Autodesk Inventor part; units mm, degrees
(part 2 of 2)
sketch "Sketch8" plane through (0, 0, 0) normal (0, 0, -1) x (-1, 0, 0)
  circle A0 centre (-9.222618, -23.066498) radius 1.25
  arc A1 (-6.852288, -24.648912) -> (-5.454999, -24.922583) centre (-5.454876, -21.21803) ccw
  arc A2 (-7.079113, -24.944764) -> (-6.852288, -24.648912) centre (-9.222618, -23.066498) ccw
  arc A3 (-6.452085, -26.223102) -> (-7.079113, -24.944764) centre (-10.029598, -27.184931) ccw
  arc A4 (-6.887807, -26.557724) -> (-6.452085, -26.223102) centre (-9.222618, -23.066498) ccw
  arc A5 (-7.961059, -25.622074) -> (-6.887807, -26.557724) centre (-5.035423, -23.349549) ccw
  arc A6 (-8.305421, -25.764877) -> (-7.961059, -25.622074) centre (-9.222618, -23.066498) ccw
  arc A7 (-8.401568, -27.185463) -> (-8.305421, -25.764877) centre (-11.9807, -26.229676) ccw
  arc A8 (-8.946225, -27.257393) -> (-8.401568, -27.185463) centre (-9.222618, -23.066498) ccw
  arc A9 (-9.407864, -25.910471) -> (-8.946225, -27.257393) centre (-5.737927, -25.405224) ccw
  arc A10 (-9.777492, -25.861961) -> (-9.407864, -25.910471) centre (-9.222618, -23.066498) ccw
  arc A11 (-10.571051, -27.044151) -> (-9.777492, -25.861961) centre (-13.192776, -24.42685) ccw
  arc A12 (-11.078703, -26.834116) -> (-10.571051, -27.044151) centre (-9.222618, -23.066498) ccw
  arc A13 (-10.805032, -25.436828) -> (-11.078703, -26.834116) centre (-7.37415, -26.83424) ccw
  arc A14 (-11.100884, -25.210003) -> (-10.805032, -25.436828) centre (-9.222618, -23.066498) ccw
  arc A15 (-12.379222, -25.83703) -> (-11.100884, -25.210003) centre (-13.341052, -22.259518) ccw
  arc A16 (-12.713844, -25.401308) -> (-12.379222, -25.83703) centre (-9.222618, -23.066498) ccw
  arc A17 (-11.778194, -24.328057) -> (-12.713844, -25.401308) centre (-9.505669, -27.253692) ccw
  arc A18 (-11.920997, -23.983694) -> (-11.778194, -24.328057) centre (-9.222618, -23.066498) ccw
  arc A19 (-13.341583, -23.887547) -> (-11.920997, -23.983694) centre (-12.385796, -20.308416) ccw
  arc A20 (-13.413513, -23.34289) -> (-13.341583, -23.887547) centre (-9.222618, -23.066498) ccw
  arc A21 (-12.066591, -22.881252) -> (-13.413513, -23.34289) centre (-11.561344, -26.551189) ccw
  arc A22 (-12.018081, -22.511624) -> (-12.066591, -22.881252) centre (-9.222618, -23.066498) ccw
  arc A23 (-13.200271, -21.718065) -> (-12.018081, -22.511624) centre (-10.58297, -19.096339) ccw
  arc A24 (-12.990236, -21.210413) -> (-13.200271, -21.718065) centre (-9.222618, -23.066498) ccw
  arc A25 (-11.592948, -21.484083) -> (-12.990236, -21.210413) centre (-12.99036, -24.914965) ccw
  arc A26 (-11.366123, -21.188231) -> (-11.592948, -21.484083) centre (-9.222618, -23.066498) ccw
  arc A27 (-11.99315, -19.909894) -> (-11.366123, -21.188231) centre (-8.415638, -18.948064) ccw
  arc A28 (-11.557428, -19.575272) -> (-11.99315, -19.909894) centre (-9.222618, -23.066498) ccw
  arc A29 (-10.484177, -20.510922) -> (-11.557428, -19.575272) centre (-13.409812, -22.783446) ccw
  arc A30 (-10.139814, -20.368118) -> (-10.484177, -20.510922) centre (-9.222618, -23.066498) ccw
  arc A31 (-10.043667, -18.947532) -> (-10.139814, -20.368118) centre (-6.464536, -19.903319) ccw
  arc A32 (-9.49901, -18.875602) -> (-10.043667, -18.947532) centre (-9.222618, -23.066498) ccw
  arc A33 (-9.037372, -20.222524) -> (-9.49901, -18.875602) centre (-12.707309, -20.727771) ccw
  arc A34 (-8.667744, -20.271034) -> (-9.037372, -20.222524) centre (-9.222618, -23.066498) ccw
  arc A35 (-7.874185, -19.088844) -> (-8.667744, -20.271034) centre (-5.252459, -21.706146) ccw
  arc A36 (-7.366533, -19.298879) -> (-7.874185, -19.088844) centre (-9.222618, -23.066498) ccw
  arc A37 (-7.640203, -20.696167) -> (-7.366533, -19.298879) centre (-11.071085, -19.298755) ccw
  arc A38 (-7.344351, -20.922993) -> (-7.640203, -20.696167) centre (-9.222618, -23.066498) ccw
  arc A39 (-6.066014, -20.295965) -> (-7.344351, -20.922993) centre (-5.104184, -23.873478) ccw
  arc A40 (-5.731392, -20.731687) -> (-6.066014, -20.295965) centre (-9.222618, -23.066498) ccw
  arc A41 (-6.667042, -21.804939) -> (-5.731392, -20.731687) centre (-8.939567, -18.879303) ccw
  arc A42 (-6.524238, -22.149301) -> (-6.667042, -21.804939) centre (-9.222618, -23.066498) ccw
  arc A43 (-5.103652, -22.245448) -> (-6.524238, -22.149301) centre (-6.059439, -25.82458) ccw
  arc A44 (-5.031722, -22.790105) -> (-5.103652, -22.245448) centre (-9.222618, -23.066498) ccw
  arc A45 (-6.378644, -23.251744) -> (-5.031722, -22.790105) centre (-6.883891, -19.581807) ccw
  arc A46 (-6.427154, -23.621372) -> (-6.378644, -23.251744) centre (-9.222618, -23.066498) ccw
  arc A47 (-5.244964, -24.414931) -> (-6.427154, -23.621372) centre (-7.862266, -27.036656) ccw
  arc A48 (-5.454999, -24.922583) -> (-5.244964, -24.414931) centre (-9.222618, -23.066498) ccw
  circle A49 centre (-9.222618, -23.066498) radius 4.2
  circle A50 centre (-9.222618, -23.066498) radius 4.6
  point P0 (0, 0)
  dimension "d138" = 0.4
  constraints: 1 centre point, 1 coincident, 3 other
extrude "Extrusion10" add sketch "Sketch8" against normal blind 1.6 contours A2 A3 A4 A5 A6 A7 A8 A9 A10 A11 A12 A13 A14 A15 A16 A17 A18 A19 A20 A21 A22 A23 A24 A25 A26 A27 A28 A29 A30 A31 A32 A33 A34 A35 A36 A37 A38 A39 A40 A41 A42 A43 A44 A45 A46 A47 A48 A1 | A1 A49 A3 A2 | A47 A46 A45 A49 | A49 A7 A6 A5 | A43 A42 A41 A49 | A49 A11 A10 A9 | A39 A38 A37 A49 | A49 A15 A14 A13 | A35 A34 A33 A49 | A49 A19 A18 A17 | A31 A30 A29 A49 | A49 A23 A22 A21 | A27 A26 A25 A49 | A50
fillet "Fillet1" radius 1 5 edges at (1.9609, -60.1053, 2) (5.9625, -57.7949, 2) (8.4625, -62.125, 2) (4.4609, -64.4354, 2) (20.9375, -49.1491, 2)
sketch "Sketch10" plane through (0, 0, 9.3) normal (0, 0, 1) x (1, 0, 0)
  arc A0 (2, -23.367949) -> (-1, -25.1) centre (1, -25.1) ccw
  line L0 (-1, -33.180447) -> (-1, -25.1)
  spline S0 degree 2 poles (-1, -33.180447) (0.437273, -35.168536) (-1, -37.156626) knots 0 0 0 1 1 1 weights 1 1.44736842 1 construction
  line L1 (-1, -45.237072) -> (-1, -37.156626)
  line L2 (23.1, -65.837072) -> (0, -65.837072)
  line L3 (23.1, -6.5) -> (23.1, -65.837072)
  line L4 (27.4, -6.5) -> (23.1, -6.5)
  line L5 (27.4, 0) -> (27.4, -6.5)
  line L6 (0, 0) -> (27.4, 0)
  line L7 (0, -1) -> (0, 0)
  line L8 (2.5, -1) -> (0, -1)
  line L9 (2.5, -17.5) -> (2.5, -1)
  line L10 (0, -17.5) -> (2.5, -17.5)
  line L11 (0, -65.837072) -> (0, -17.5)
  arc A1 (4.054242, -29.688272) -> (16.938443, -26.387046) centre (12.35, -35.272213) ccw
  arc A2 (9.70004, -14.680076) -> (4.054242, -29.688272) centre (9.222618, -23.066498) ccw
  arc A3 (16.718073, -19.274645) -> (9.70004, -14.680076) centre (14.7, -14.7) ccw
  arc A4 (16.938443, -26.387046) -> (16.718073, -19.274645) centre (9.222618, -23.066498) ccw
  circle A5 centre (1.4, -30.091255) radius 0.6
  circle A6 centre (1.4, -41.171175) radius 0.6
  circle A7 centre (1.4, -30.091255) radius 2.113828
  circle A8 centre (1.4, -41.171175) radius 2.437856
  circle A9 centre (4, -46.509539) radius 3.5
  arc A10 (4.054242, -29.688272) -> (16.938443, -26.387046) centre (12.35, -35.272213) ccw
  arc A11 (9.70004, -14.680076) -> (4.054242, -29.688272) centre (9.222618, -23.066498) ccw
  circle A12 centre (9.043146, -9.043146) radius 2.25
  circle A13 centre (20.356854, -20.356854) radius 2.25
  arc A14 (-1, -45.237072) -> (2, -46.969123) centre (1, -45.237072) ccw
  spline S1 degree 3 poles (3, -25.1) (3, -24.918932) (2.974149, -24.721818) (2.859633, -24.337077) (2.770851, -24.149343) (2.583999, -23.871436) (2.486925, -23.753405) (2.26049, -23.539413) (2.130887, -23.443517) (2, -23.367949) knots 0 0 0 0 0.29735014 0.29735014 0.59470027 0.59470027 0.79735014 0.79735014 1 1 1 1
  spline S2 degree 3 poles (2, -46.969123) (2.144805, -46.88552) (2.285887, -46.778364) (2.528279, -46.538397) (2.629848, -46.405654) (2.897307, -45.967482) (3, -45.573174) (3, -45.237072) knots 0 0 0 0 0.2241219 0.2241219 0.4482438 0.4482438 1 1 1 1
  line L12 (3, -25.1) -> (3, -45.237072)
  circle A15 centre (4, -46.509539) radius 1.2295
  point P0 (0, 0)
  point P1 (19.495918, -28.276795)
  dimension "d145" = 1.2
  dimension "d146" = 1.2
  dimension "d147" = 4.22766
  dimension "d148" = 4.87571
  dimension "d149" = 7
  dimension "d226" = 0.8
  dimension "d227" = 1
  dimension "d228" = 0.8
  dimension "d229" = 1
  constraints: 5 centre point, 4 tangent, 3 coincident, 2 end point, 1 vertical
  measures "d145" diameter of A5
  measures "d146" diameter of A6
  measures "d147" diameter of A7
  measures "d148" diameter of A8
  measures "d149" diameter of A9
  measures "d226" distance edge to line of A5 L11
  measures "d227" distance edge to line of A5 L12
  measures "d228" distance edge to line of A6 L11
  measures "d229" distance edge to line of A6 L12
hole "Hole7" at (1.4, -30.091255, 9.3) at (1.4, -41.171175, 9.3) direction (0, 0, -1) diameter 1.4 end through all
sketch "Sketch11" plane through (2.5, -17.5, 0) normal (-1, 0, 0) x (0, 0, 1)
  circle A0 centre (6, 7) radius 1.25 projected
  point P0 (0, 17.5)
hole "Hole8" at (2.5, -10.5, 6) direction (1, 0, 0) diameter 2.013 depth 8 thread size "M2.5x0.45" class "6H" standard "ISO Metric profile"
sketch "Sketch13" plane through (0, 0, 3.1) normal (0, 0, 1) x (1, 0, 0)
  arc A0 (6.782075, -26.965696) -> (13.237489, -25.311672) centre (12.35, -35.272213) ccw
  arc A1 (6.782075, -26.965696) -> (13.237489, -25.311672) centre (9.222618, -23.066498) ccw
  circle A2 centre (12.35, -35.272213) radius 5
  circle A3 centre (14.7, -14.7) radius 14
  circle A4 centre (14.7, -55.637072) radius 14
  circle A5 centre (18.362153, -30.788463) radius 2.5
  circle A6 centre (18.490592, -39.578386) radius 2.5
  circle A7 centre (6.124853, -31.089206) radius 2.5
  circle A8 centre (7.351555, -40.863773) radius 2.5
  point P0 (0, 0)
  dimension "d174" = 5
  dimension "d175" = 5
  dimension "d176" = 5
  dimension "d177" = 5
  dimension "d178" = 1.5
  constraints: 7 tangent, 4 centre point
  measures "d174" diameter of A5
  measures "d175" diameter of A6
  measures "d176" diameter of A8
  measures "d177" diameter of A7
hole "Hole10" at (18.362153, -30.788463, 3.1) at (18.490592, -39.578386, 3.1) at (7.351555, -40.863773, 3.1) at (6.124853, -31.089206, 3.1) direction (0, 0, -1) diameter 2.9 end through all counterbore diameter 5 counterbore depth 1.1 clearance for "Countersunk Flat Head Screw ISO 2009/7046" size "M2.5" standard "ISO"
sketch "Sketch14" plane through (0, 0, 3.1) normal (0, 0, 1) x (1, 0, 0)
  arc A0 (8.199902, -32.483542) -> (4.049804, -29.694871) centre (6.124853, -31.089206) ccw
  arc A1 (16.358102, -32.283046) -> (8.199902, -32.483542) centre (12.35, -35.272213) ccw
  arc A2 (20.366204, -29.293879) -> (16.358102, -32.283046) centre (18.362153, -30.788463) ccw
  arc A3 (20.366204, -29.293879) -> (13.237489, -25.311672) centre (12.35, -35.272213) ccw
  arc A4 (6.782075, -26.965696) -> (13.237489, -25.311672) centre (9.222618, -23.066498) ccw
  arc A5 (6.782075, -26.965696) -> (4.049804, -29.694871) centre (12.35, -35.272213) ccw
  arc A6 (20.537456, -41.013777) -> (16.443728, -38.142995) centre (18.490592, -39.578386) ccw
  arc A7 (20.537456, -41.013777) -> (20.366204, -29.293879) centre (12.35, -35.272213) ccw
  arc A8 (16.358102, -32.283046) -> (20.366204, -29.293879) centre (18.362153, -30.788463) ccw
  arc A9 (16.443728, -38.142995) -> (16.358102, -32.283046) centre (12.35, -35.272213) ccw
  arc A10 (5.685407, -42.727627) -> (9.017703, -38.99992) centre (7.351555, -40.863773) ccw
  arc A11 (5.685407, -42.727627) -> (20.537456, -41.013777) centre (12.35, -35.272213) ccw
  arc A12 (16.443728, -38.142995) -> (20.537456, -41.013777) centre (18.490592, -39.578386) ccw
  arc A13 (9.017703, -38.99992) -> (16.443728, -38.142995) centre (12.35, -35.272213) ccw
  arc A14 (4.049804, -29.694871) -> (8.199902, -32.483542) centre (6.124853, -31.089206) ccw
  arc A15 (4.049804, -29.694871) -> (5.685407, -42.727627) centre (12.35, -35.272213) ccw
  arc A16 (9.017703, -38.99992) -> (5.685407, -42.727627) centre (7.351555, -40.863773) ccw
  arc A17 (8.199902, -32.483542) -> (9.017703, -38.99992) centre (12.35, -35.272213) ccw
  line L0 (16.28503, -29.39722) -> (15.132486, -31.117965)
  line L1 (19.103243, -33.176095) -> (17.125264, -33.790033)
  line L2 (15.252677, -39.343388) -> (16.455005, -41.029724)
  circle A18 centre (12.35, -35.272213) radius 5
  line L3 (10.45085, -39.897494) -> (9.664196, -41.813348)
  line L4 (7.965712, -37.675963) -> (6.14968, -38.671629)
  line L5 (9.366807, -31.259662) -> (8.131128, -29.59761)
  line L6 (5.501944, -33.51036) -> (7.507693, -34.026395)
  line L7 (17.166531, -36.614236) -> (19.161604, -37.17012)
  arc A19 (4.049804, -29.694871) -> (8.199902, -32.483542) centre (6.124853, -31.089206) ccw
  arc A20 (8.199902, -32.483542) -> (4.049804, -29.694871) centre (6.124853, -31.089206) ccw
  arc A21 (9.017703, -38.99992) -> (5.685407, -42.727627) centre (7.351555, -40.863773) ccw
  arc A22 (5.685407, -42.727627) -> (9.017703, -38.99992) centre (7.351555, -40.863773) ccw
  arc A23 (9.017703, -38.99992) -> (16.443728, -38.142995) centre (12.35, -35.272213) ccw
  arc A24 (16.443728, -38.142995) -> (20.537456, -41.013777) centre (18.490592, -39.578386) ccw
  arc A25 (16.358102, -32.283046) -> (20.366204, -29.293879) centre (18.362153, -30.788463) ccw
  arc A26 (16.358102, -32.283046) -> (8.199902, -32.483542) centre (12.35, -35.272213) ccw
  point P0 (0, 0)
  point P1 (16.358102, -32.283046)
  point P2 (16.358102, -32.283046)
  point P3 (16.358102, -32.283046)
  point P4 (16.358102, -32.283046)
  point P5 (16.443728, -38.142995)
  point P6 (16.443728, -38.142995)
  point P7 (16.443728, -38.142995)
  point P8 (16.443728, -38.142995)
  constraints: 18 point on circle, 16 end point, 8 tangent, 2 line through centre, 12 other
extrude "Extrusion12" cut sketch "Sketch14" against normal up to surface (1.1 mm away) contours A0 L5 A1 | A17 L6 A14 | L0 A2 A1 | A17 A16 L4 | A8 L1 A9 | A13 L3 A10 | A6 A9 L7 | L2 A13 A12
sketch "Sketch15" plane through (0, 0, 0) normal (0, 1, 0) x (1, 0, 0)
  line L0 (27.4, 0) -> (0, 0) projected
  line L1 (0, 0) -> (0, -9.3) projected
  line L2 (0, -9.3) -> (27.4, -9.3) projected
  line L3 (27.4, 0) -> (27.4, -9.3) projected
  line L4 (27.4, 0) -> (0, 0) projected
  line L5 (23.1, 0) -> (23.1, -9.3)
  line L6 (3, -9.3) -> (3, 0)
  line L7 (0, 0) -> (0, -9.3) projected
  circle A0 centre (18.075, -3.25) radius 3.25
  circle A1 centre (8.025, -3.25) radius 3.25
  line L8 (13.05, 0) -> (13.05, -9.3)
  dimension "d195" = 4.3
  dimension "d196" = 3
  dimension "d197" = 6.5
  dimension "d198" = 6.5
  dimension "d202" = 5.025
  dimension "d203" = 5.025
  dimension "d206" = 10.05
  dimension "d207" = 10.05
  dimension "d208" = 5.025
  dimension "d209" = 5.025
  constraints: 6 end point, 6 point on line, 2 centre point, 2 perpendicular, 2 tangent, 1 parallel
  measures "d195" distance between parallel lines of L3 L5
  measures "d196" distance between parallel lines of L1 L6
  measures "d197" diameter of A0
  measures "d198" diameter of A1
  measures "d202" distance from line of A0.centre L5
  measures "d203" distance from line of L6 A1.centre
  measures "d206" distance between parallel lines of L6 L8
  measures "d207" distance between parallel lines of L5 L8
  measures "d208" distance from line of L8 A0.centre
  measures "d209" distance from line of A1.centre L8
hole "Hole11" at (18.075, 0, 3.25) at (8.025, 0, 3.25) direction (0, -1, 0) diameter 2.459 depth 6.5 thread size "M3x0.5" class "6H" standard "ISO Metric profile"
ref_plane "Work Plane4" through (0, 1, 0) normal (0, 1, 0) x (1, 0, 0)
sketch "Sketch16" plane through (0, 1, 0) normal (0, 1, 0) x (1, 0, 0)
  circle A0 centre (18.075, -3.25) radius 1.2295 projected
  circle A1 centre (8.025, -3.25) radius 1.2295 projected
  point P0 (0, 0)
hole "Hole12" at (8.025, 1, 3.25) at (18.075, 1, 3.25) direction (0, -1, 0) diameter 0.1 depth 5 countersink diameter 7 countersink angle 90
fillet "Fillet2" radius 1 8 edges at (15.2527, -39.3434, 2.55) (17.1665, -36.6142, 2.55) (10.4508, -39.8975, 2.55) (7.9657, -37.676, 2.55) (7.5077, -34.0264, 2.55) (15.1325, -31.118, 2.55) (17.1253, -33.79, 2.55) (9.3668, -31.2597, 2.55)
body "Solid2"
